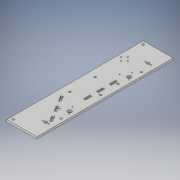
# Autodesk Inventor part: ChassisOutide10
Saved by Autodesk Inventor 2019 (Build 230136000, 136)
## iProperties
Created: 2019-10-11
Part Number: ChassisOutide10
Material: Generic
Document SubType Name: Modeling
Designer: shrey
Density: 1 g/cm^3
Appearance: Default
Author: shrey
Autodesk Inventor part; units mm, degrees
ref_plane "YZ Plane" through (0, 0, 0) normal (1, 0, 0) x (0, 1, 0)
ref_plane "XZ Plane" through (0, 0, 0) normal (0, 1, 0) x (-1, 0, 0)
ref_plane "XY Plane" through (0, 0, 0) normal (0, 0, 1) x (1, 0, 0)
sketch "Sketch1" plane through (0, 0, 0) normal (0, 1, 0) x (-1, 0, 0)
  line L0 (44.45, 203.2) -> (-44.45, 203.2)
  line L1 (-44.45, 203.2) -> (-44.45, -203.2)
  line L2 (-44.45, -203.2) -> (44.45, -203.2)
  line L3 (44.45, -203.2) -> (44.45, 203.2)
  line L4 (44.45, 203.2) -> (-44.45, -203.2) construction
  line L5 (-44.45, 203.2) -> (44.45, -203.2) construction
  line L6 (-44.45, 203.2) -> (-20.955, 203.2)
  line L7 (-20.955, 203.2) -> (-20.955, 88.9) construction
  line L8 (-44.45, 88.9) -> (-44.45, 203.2)
  circle A0 centre (-20.955, 88.9) radius 15.494 construction
  line L9 (44.45, 203.2) -> (44.45, 111.6492)
  line L10 (44.45, 203.2) -> (44.45, 38.1)
  line L11 (44.45, 38.1) -> (22.225, 38.1) construction
  circle A1 centre (22.225, 38.1) radius 12.065 construction
  line L12 (-66.675, 88.9) -> (0, 88.9) construction
  line L13 (0, 88.9) -> (0, 203.2) construction
  line L14 (0, 203.2) -> (-66.675, 203.2)
  line L15 (-66.675, 203.2) -> (-66.675, 88.9) construction
  line L16 (-66.675, 203.2) -> (-66.675, 209.55) construction
  line L17 (-66.675, 209.55) -> (32.5679, 44.312) construction
  circle A2 centre (-20.955, 104.394) radius 1.5
  circle A3 centre (-34.3732, 96.647) radius 1.5
  circle A4 centre (-34.3732, 81.153) radius 1.5
  circle A5 centre (-20.955, 73.406) radius 1.5
  circle A6 centre (-7.5368, 81.153) radius 1.5
  circle A7 centre (-7.5368, 96.647) radius 1.5
  circle A8 centre (-20.955, 88.9) radius 7.112 construction
  circle A9 centre (-28.067, 88.9) radius 5.9944
  line L18 (-20.955, 88.9) -> (-20.955, 152.4) construction
  circle A10 centre (-20.955, 152.4) radius 8.001 construction
  circle A11 centre (-20.955, 152.4) radius 4.0005
  circle A12 centre (-20.955, 160.401) radius 1.85
  line L19 (42.545, 152.4) -> (-20.955, 152.4) construction
  circle A13 centre (-28.956, 152.4) radius 1.85
  line L20 (-20.955, 215.9) -> (-20.955, 152.4) construction
  circle A14 centre (-20.955, 144.399) radius 1.85
  line L21 (-84.455, 152.4) -> (-20.955, 152.4) construction
  circle A15 centre (-12.954, 152.4) radius 1.85
  line L22 (44.45, 0) -> (-44.45, 0) construction
  circle A16 centre (22.225, 38.1) radius 2.9766
  circle A17 centre (22.225, -38.1) radius 2.9766
  circle A18 centre (-33.8743, 119.8397) radius 12.065 construction
  circle A19 centre (-33.8743, 119.8397) radius 2.9766
  circle A20 centre (-20.955, 152.4) radius 50.8 construction
  line L23 (32.5679, 44.312) -> (22.7595, 60.6429) construction
  line L24 (22.7595, 60.6429) -> (17.8553, 68.8083) construction
  line L25 (15.6729, 78.6085) -> (25.4813, 62.2776)
  line L26 (25.4813, 62.2776) -> (20.0377, 59.0081)
  line L27 (20.0377, 59.0081) -> (10.2292, 75.339)
  line L28 (10.2292, 75.339) -> (15.6729, 78.6085)
  line L29 (15.6729, 78.6085) -> (20.0377, 59.0081) construction
  line L30 (25.4813, 62.2776) -> (10.2292, 75.339) construction
  line L31 (-3.944, 111.2702) -> (5.8645, 94.9394)
  line L32 (-9.3876, 108.0008) -> (-3.944, 111.2702)
  line L33 (5.8645, 94.9394) -> (0.4208, 91.6699)
  line L34 (0.4208, 91.6699) -> (-9.3876, 108.0008)
  line L35 (-23.5608, 143.932) -> (-13.7524, 127.6011)
  line L36 (-29.0044, 140.6625) -> (-23.5608, 143.932)
  line L37 (-13.7524, 127.6011) -> (-19.196, 124.3316)
  line L38 (-19.196, 124.3316) -> (-29.0044, 140.6625)
  circle A21 centre (-20.955, -104.394) radius 1.5
  circle A22 centre (-34.3732, -81.153) radius 1.5
  circle A23 centre (-7.5368, -81.153) radius 1.5
  circle A24 centre (-28.067, -88.9) radius 5.9944
  circle A25 centre (-20.955, -152.4) radius 4.0005
  circle A26 centre (-28.956, -152.4) radius 1.85
  circle A27 centre (-12.954, -152.4) radius 1.85
  circle A28 centre (22.225, -38.1) radius 2.9766
  circle A29 centre (-33.8743, -119.8397) radius 2.9766
  circle A30 centre (-29.2932, -53.9743) radius 3.175
  circle A31 centre (-28.067, 88.9) radius 31.75 construction
  line L39 (-28.067, 88.9) -> (-44.45, 88.9) construction
  line L40 (-44.45, 88.9) -> (-44.45, 12.7)
  line L41 (44.45, 203.2) -> (34.925, 203.2)
  line L42 (34.925, 203.2) -> (34.925, 193.675) construction
  line L43 (34.925, 193.675) -> (44.45, 193.675) construction
  line L44 (44.45, 193.675) -> (44.45, 203.2)
  circle A32 centre (34.925, 193.675) radius 3.175
  line L45 (-44.45, 0) -> (-31.75, 0)
  circle A33 centre (-31.75, 0) radius 3.175
  circle A34 centre (34.925, -193.675) radius 3.175
  line L46 (-44.45, 0) -> (-19.455, 0) construction
  line L47 (-16.28, -76.0639) -> (-22.63, -76.0639) construction
  line L48 (-22.63, -76.0639) -> (-22.63, 51.9267) construction
  line L49 (-22.63, 51.9267) -> (-16.28, 51.9267) construction
  line L50 (-16.28, 51.9267) -> (-16.28, -76.0639) construction
  line L51 (-16.28, -63.9953) -> (-22.63, 63.9953) construction
  line L52 (-22.63, -63.9953) -> (-16.28, 63.9953) construction
  line L53 (-16.28, 51.9267) -> (-22.63, -76.0639) construction
  line L54 (-22.63, 51.9267) -> (-16.28, -76.0639) construction
  line L55 (-16.28, -2.5436) -> (-22.63, -2.5436)
  line L56 (-22.63, -2.5436) -> (-22.63, -21.5936)
  line L57 (-22.63, -21.5936) -> (-16.28, -21.5936)
  line L58 (-16.28, -21.5936) -> (-16.28, -2.5436)
  line L59 (-16.28, -2.5436) -> (-22.63, -21.5936) construction
  line L60 (-22.63, -2.5436) -> (-16.28, -21.5936) construction
  line L61 (-16.28, -40.6436) -> (-22.63, -40.6436)
  line L62 (-16.28, -59.6936) -> (-16.28, -40.6436)
  line L63 (-22.63, -40.6436) -> (-22.63, -59.6936)
  line L64 (-22.63, -59.6936) -> (-16.28, -59.6936)
  line L65 (-16.28, 35.5564) -> (-22.63, 35.5564)
  line L66 (-16.28, 16.5064) -> (-16.28, 35.5564)
  line L67 (-22.63, 35.5564) -> (-22.63, 16.5064)
  line L68 (-22.63, 16.5064) -> (-16.28, 16.5064)
  line L69 (-16.28, -2.5436) -> (-22.63, -2.5436)
  line L70 (-16.28, -21.5936) -> (-16.28, -2.5436)
  line L71 (-22.63, -2.5436) -> (-22.63, -21.5936)
  line L72 (-22.63, -21.5936) -> (-16.28, -21.5936)
  line L73 (44.45, -203.2) -> (25.4, -203.2)
  line L74 (25.4, -203.2) -> (25.4, -128.2) construction
  line L75 (25.4, -128.2) -> (44.45, -128.2) construction
  line L76 (44.45, -128.2) -> (44.45, -203.2)
  circle A35 centre (25.4, -128.2) radius 6.35 construction
  circle A36 centre (25.4, -128.2) radius 9.779 construction
  circle A37 centre (15.621, -128.2) radius 1.778
  circle A38 centre (25.4, -128.2) radius 6.35 construction
  circle A39 centre (25.4, -128.2) radius 9.779 construction
  line L77 (100.4, -128.2) -> (25.4, -128.2) construction
  line L78 (25.4, -128.2) -> (25.4, -109.15) construction
  circle A40 centre (25.4, -137.979) radius 1.778
  circle A41 centre (25.4, -128.2) radius 6.35 construction
  circle A42 centre (25.4, -128.2) radius 9.779 construction
  line L79 (25.4, -53.2) -> (25.4, -128.2) construction
  line L80 (25.4, -128.2) -> (6.35, -128.2) construction
  circle A43 centre (35.179, -128.2) radius 1.778
  circle A44 centre (25.4, -128.2) radius 6.35 construction
  circle A45 centre (25.4, -128.2) radius 9.779 construction
  line L81 (-49.6, -128.2) -> (25.4, -128.2) construction
  line L82 (25.4, -128.2) -> (25.4, -147.25) construction
  circle A46 centre (25.4, -118.421) radius 1.778
  point P0 (0, 0)
  point P1 (-19.455, -12.0686)
  dimension "d4" = 30.988
  dimension "d7" = 24.13
  dimension "d16" = 14.224
  dimension "d19" = 16.002
  dimension "d74" = 19.558
  dimension "d0" = 88.9
  dimension "d1" = 406.4
  dimension "d2" = 114.3
  dimension "d3" = 23.495
  dimension "d5" = 165.1
  dimension "d6" = 22.225
  dimension "d10" = 6.35
  dimension "d14" = 360
  dimension "d17" = 11.9888
  dimension "d18" = 63.5
  dimension "d20" = 8.001
  dimension "d21" = 3.7
  dimension "d24" = 360
  dimension "d26" = 5.9531
  dimension "d27" = 24.13
  dimension "d28" = 5.9531
  dimension "d29" = 101.6
  dimension "d32" = 19.05
  dimension "d33" = 9.525
  dimension "d34" = 6.35
  dimension "d37" = 38.1
  dimension "d48" = 63.5
  dimension "d50" = 9.525
  dimension "d51" = 9.525
  dimension "d52" = 6.35
  dimension "d53" = 12.7
  dimension "d54" = 6.35
  dimension "d57" = 6.35
  dimension "d58" = 127.9906
  dimension "d59" = 6.35
  dimension "d60" = 19.05
  dimension "d63" = 38.1
  dimension "d66" = 38.1
  dimension "d71" = 75
  dimension "d72" = 19.05
  dimension "d73" = 12.7
  dimension "d75" = 3.556
  dimension "d78" = 360
  constraints: 166 end point, 39 centre point, 20 coincident, 17 parallel, 12 midpoint, 11 symmetric about line, 10 point on line, 9 horizontal, 9 perpendicular, 4 vertical alignment, 3 horizontal alignment, 3 vertical, 1 collinear, 146 other
  measures "d0" distance of L1.end L2.end
  measures "d1" distance of L0.end L1.end
  measures "d2" distance of L6.end L7.end
  measures "d3" distance of L7.end L8.start
  measures "d5" distance of L0.start L10.end
  measures "d6" distance of L10.end L11.end
  measures "d10" distance of L14.end L16.end
  measures "d17" diameter of A9
  measures "d18" distance of L18.start L18.end
  measures "d20" diameter of A11
  measures "d21" diameter of A12
  measures "d26" diameter of A16
  measures "d27" diameter of A18
  measures "d28" diameter of A19
  measures "d29" diameter of A20
  measures "d32" distance of L17.end L23.end
  measures "d33" distance of L23.end L24.end
  measures "d34" distance of L25.end L26.end
  measures "d37" distance of L25.start L31.start
  measures "d48" diameter of A31
  measures "d50" distance of L42.end L43.end
  measures "d51" distance of L41.end L42.end
  measures "d52" diameter of A32
  measures "d53" distance of L22.end L45.end
  measures "d54" diameter of A33
  measures "d57" distance of L48.end L49.end
  measures "d58" distance of L47.end L48.end
  measures "d59" distance of L57.end L56.end
  measures "d60" distance of L56.end L55.end
  measures "d63" distance of L55.start L61.start
  measures "d66" distance of L55.start L65.start
  measures "d71" distance of L73.end L74.end
  measures "d72" distance of L74.end L75.end
  measures "d73" diameter of A35
  measures "d75" diameter of A37
extrude "Extrusion6" add sketch "Sketch1" along normal blind 6.35 contours L3 L2 L1 L0 | A2 | A4 | A6 | A12 | A14
body "Solid6"
